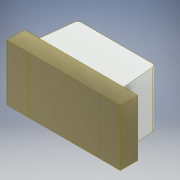
# Autodesk Inventor part: LED_1608
Saved by Autodesk Inventor 2017 (Build 210142000, 142)
## iProperties
Created: 2018-05-13
Part Number: LED_1608
Material: ABS Plastic
Document SubType Name: Modeling
Designer: Bradley
Density: 1.06 g/cm^3
Appearance: Gold - Metal
Author: Bradley
Autodesk Inventor part; units mm, degrees
ref_plane "YZ Plane" through (0, 0, 0) normal (1, 0, 0) x (0, 1, 0)
ref_plane "XZ Plane" through (0, 0, 0) normal (0, 1, 0) x (-1, 0, 0)
ref_plane "XY Plane" through (0, 0, 0) normal (0, 0, 1) x (1, 0, 0)
sketch "Sketch1" plane through (0, 0, 0) normal (0, 0, 1) x (1, 0, 0)
  line L0 (1.1, -0.25) -> (0.1, -0.25)
  line L1 (1.1, -0.25) -> (1.1, -0.2501)
  line L2 (1.401, -0.2501) -> (1.1, -0.2501)
  line L3 (1.401, 0.0001) -> (1.401, -0.2501)
  line L4 (1.2, 0.0001) -> (1.401, 0.0001)
  line L5 (1.2, 0) -> (1.2, 0.0001)
  line L6 (1.2, 0) -> (0, 0)
  line L7 (0, 0) -> (0, 0.0001)
  line L8 (0, 0.0001) -> (-0.2, 0.0001)
  line L9 (-0.2, 0) -> (-0.2, 0.0001)
  line L10 (-0.21, 0) -> (-0.2, 0)
  line L11 (-0.21, -0.25) -> (-0.21, 0)
  line L12 (-0.21, -0.25) -> (-0.2, -0.25)
  line L13 (-0.2, -0.25) -> (-0.2, -0.2501)
  line L14 (0.1, -0.2501) -> (-0.2, -0.2501)
  line L15 (0.1, -0.25) -> (0.1, -0.2501)
  line L16 (0.0952, 0.5) -> (1.1048, 0.5)
  arc A0 (0.0952, 0.5) -> (0.0455, 0.455) centre (0.0952, 0.45) ccw
  line L17 (0, 0) -> (0.0455, 0.455)
  line L18 (1.2, 0) -> (0, 0)
  line L19 (1.1545, 0.455) -> (1.2, 0)
  arc A1 (1.1545, 0.455) -> (1.1048, 0.5) centre (1.1048, 0.45) ccw
  point P0 (0.6, -0.125)
  constraints: 40 end point, 10 horizontal, 8 vertical, 4 point on circle, 2 centre point, 30 other
extrude "Extrusion1" add sketch "Sketch1" along normal mid plane 0.8 contours L0 L14 L12 L11 L10 L8 L6 L4 L3 L2
extrude "Extrusion2" add sketch "Sketch1" along normal mid plane 0.79 contours L6 L17 A0 L16 A1 L19
body "Solid1"
